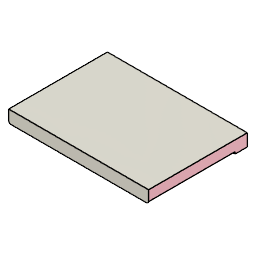
minecraft_pig (Autodesk Fusion 360 archive; units mm, degrees)
design "Bottom Face Plate"
part number: 2025-10-08-20-58-30-384
Autodesk Fusion 360 part; units mm, degrees
sketch "Bottom Face Plate" plane through (0, 0, 0) normal (0, 0, 1) x (1, 0, 0)
  line L0 (0, 0) -> (136, 0)
  line L1 (136, 0) -> (136, 96)
  line L2 (136, 96) -> (0, 96)
  line L3 (0, 96) -> (0, 0)
  dimension "d5" = 136
  dimension "d6" = 96
  constraint horizontal L0
  constraint vertical L1
  constraint horizontal L2
  constraint vertical L3
  constraint coincident L0.start L3.end
  measures "d5" distance of L0.start L0.end
  measures "d6" distance of L0.start L2.end
extrude "Extrude1" add sketch "Bottom Face Plate" along normal blind 12 makes body 1
ref_plane "WorkPlane1" through (68, 84, 6) normal (0, 1, 0) x (-1, 0, 0)
split "Split1" by plane through (68, 84, 6) normal (0, 1, 0) bodies 1 makes body 2 at (90.6667, 96, 8)
fillet "Fillet1" radius 2 2 edges at (136, 42, 0) (0, 42, 0) on bodies 1
combine "Combine2" operation add target body 1 tool bodies 2
equation "block_size = 16 mm" comment "The size of the blocks used for the dimensions of the Minecraft Pig."
equation "pine_thickness = 12 mm" comment "The thickness of the pine boards used for the Minecraft Pig's body."
equation "bottom_face_plate_length = 6 * block_size" comment "The length of the Bottom Face Plate that makes up the Minecraft Pig's face."
equation "bottom_face_plate_width = 10 * block_size - 2 * pine_thickness" comment "The width of the Bottom Face Plate that makes up the Minecraft Pig's face."
equation "d5 = bottom_face_plate_width"
equation "d6 = bottom_face_plate_length"
equation "d7 = pine_thickness"
equation "d9 = -pine_thickness"
equation "fillet_radius = 2 mm" comment "The radius of the fillets applied to the Bottom Face Plate."
equation "d12 = fillet_radius"
named bodies: "Bottom Face Plate", "Bottom Face Plate (1)"

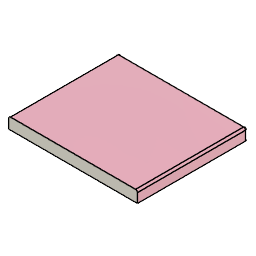
design "Top Face Plate"
part number: 2025-10-08-20-58-30-384
Autodesk Fusion 360 part; units mm, degrees
sketch "Top Face Plate" plane through (0, 0, 0) normal (0, 0, 1) x (1, 0, 0)
  line L0 (0, 0) -> (136, 0)
  line L1 (136, 0) -> (136, 116)
  line L2 (136, 116) -> (0, 116)
  line L3 (0, 116) -> (0, 0)
  dimension "d5" = 136
  dimension "d6" = 116
  constraint horizontal L0
  constraint vertical L1
  constraint horizontal L2
  constraint vertical L3
  constraint coincident L0.start L3.end
  measures "d5" distance of L0.start L0.end
  measures "d6" distance of L0.start L2.end
extrude "Extrude1" add sketch "Top Face Plate" along normal blind 12
fillet "Fillet1" radius 2 5 edges at (0, 58, 12) (136, 58, 12) (68, 116, 12) (136, 116, 6) (0, 116, 6)
equation "block_size = 16 mm" comment "The size of the blocks used for the dimensions of the Minecraft Pig."
equation "pine_thickness = 12 mm" comment "The thickness of the pine boards used for the Minecraft Pig's body."
equation "top_face_plate_length = 8 * block_size - pine_thickness" comment "The length of the Top Face Plate that makes up the Minecraft Pig's face."
equation "top_face_plate_width = 10 * block_size - 2 * pine_thickness" comment "The width of the Top Face Plate that makes up the Minecraft Pig's face."
equation "d5 = top_face_plate_width"
equation "d6 = top_face_plate_length"
equation "d7 = pine_thickness"
equation "fillet_radius = 2 mm" comment "The radius of the fillets applied to the Top Face Plate."
equation "d11 = fillet_radius"
named bodies: "Top Face Plate"

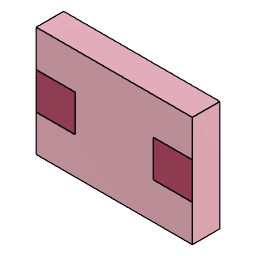
design "Nose Plate"
part number: 2025-10-11-08-44-41-819
Autodesk Fusion 360 part; units mm, degrees
sketch "Nose Plate" plane through (0, 0, 0) normal (0, 1, 0) x (1, 0, 0)
  line L0 (0, 0) -> (68, 0)
  line L1 (68, 0) -> (68, -48)
  line L2 (68, -48) -> (0, -48)
  line L3 (0, -48) -> (0, 0)
  dimension "d5" = 68
  dimension "d6" = 48
  constraint horizontal L0
  constraint vertical L1
  constraint horizontal L2
  constraint vertical L3
  constraint coincident L0.start L3.end
  measures "d5" distance of L0.start L0.end
  measures "d6" distance of L0.start L2.end
extrude "Extrude1" add sketch "Nose Plate" along normal blind 12 makes body 1
sketch "Nostrils" plane through (0, 0, 0) normal (0, -1, 0) x (1, 0, 0)
  line L0 (68, 48) -> (0, 48)
  line L1 (0, 48) -> (0, 0)
  line L2 (0, 0) -> (68, 0)
  line L3 (68, 0) -> (68, 48)
  line L4 (0, 32) -> (17, 32)
  line L5 (17, 32) -> (17, 16)
  line L6 (17, 16) -> (0, 16)
  line L7 (0, 16) -> (0, 32)
  line L8 (51, 32) -> (68, 32)
  line L9 (68, 32) -> (68, 16)
  line L10 (68, 16) -> (51, 16)
  line L11 (51, 16) -> (51, 32)
  dimension "d22" = 17
  dimension "d23" = 17
  dimension "d24" = 34
  dimension "d25" = 16
  dimension "d26" = 16
  dimension "d27" = 16
  dimension "d28" = 16
  constraint horizontal L4
  constraint vertical L5
  constraint horizontal L6
  constraint vertical L7
  constraint horizontal L8
  constraint vertical L9
  constraint horizontal L10
  constraint vertical L11
  constraint collinear L1 L7
  constraint collinear L3 L9
  measures "d22" distance of L4.start L4.end
  measures "d23" distance of L8.start L8.end
  measures "d24" distance of L5 L11
  measures "d25" distance of L4 L6
  measures "d26" distance of L8 L10
  measures "d27" distance of L0 L4
  measures "d28" distance of L0 L8
extrude "Extrude4" add sketch "Nostrils" along normal blind 0.01 separate body contours L3 L8 L9 L10 L11 | L1 L4 L5 L6 L7 makes body 2 at (5.6667, 0, 26.6667) makes body 3 at (56.6667, 0, 26.6667)
equation "block_size = 16 mm" comment "The size of the blocks used for the dimensions of the Minecraft Pig."
equation "pine_thickness = 12 mm" comment "The thickness of the pine boards used for the Minecraft Pig's body."
equation "nose_plate_height = 3 * block_size" comment "The height of the Nose Plate that makes up the Minecraft Pig's face."
equation "nose_plate_width = 4 * block_width" comment "The width of the Nose Plate that makes up the Minecraft Pig's face."
equation "d5 = nose_plate_width"
equation "d6 = nose_plate_height"
equation "d7 = pine_thickness"
equation "block_width = ( 10 * block_size - 2 * pine_thickness ) / 8" comment "The width of the blocks used for the nostrils of the Minecraft Pig."
equation "d22 = block_width"
equation "d23 = block_width"
equation "d25 = block_size"
equation "d26 = block_size"
equation "d27 = block_size"
equation "d28 = block_size"
named bodies: "Nose Plate", "Right Nostril", "Left Nostril"

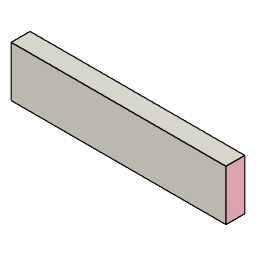
design "Back Face Plate"
part number: 2025-10-11-08-44-41-819
Autodesk Fusion 360 part; units mm, degrees
sketch "Back Face Plate" plane through (0, 0, 0) normal (0, 1, 0) x (1, 0, 0)
  line L0 (0, 0) -> (136, 0)
  line L1 (136, 0) -> (136, -32)
  line L2 (136, -32) -> (0, -32)
  line L3 (0, -32) -> (0, 0)
  dimension "d5" = 136
  dimension "d6" = 32
  constraint horizontal L0
  constraint vertical L1
  constraint horizontal L2
  constraint vertical L3
  constraint coincident L0.start L3.end
  measures "d5" distance of L0.start L0.end
  measures "d6" distance of L0.start L2.end
extrude "Extrude1" add sketch "Back Face Plate" along normal blind 12
equation "block_size = 16 mm" comment "The size of the blocks used for the dimensions of the Minecraft Pig."
equation "pine_thickness = 12 mm" comment "The thickness of the pine boards used for the Minecraft Pig's body."
equation "back_face_plate_height = 2 * block_size" comment "The height of the Back Face Plate that makes up the Minecraft Pig's face."
equation "back_face_plate_width = 10 * block_size - 2 * pine_thickness" comment "The width of the Back Face Plate that makes up the Minecraft Pig's face."
equation "d5 = back_face_plate_width"
equation "d6 = back_face_plate_height"
equation "d7 = pine_thickness"
equation "block_width = front_face_plate_width / 8" comment "The width of the blocks to use for the eyes of the Minecraft Pig."
equation "d10 = block_width"
equation "d11 = block_width"
equation "d12 = block_width"
equation "d13 = block_width"
equation "d14 = block_size"
equation "d15 = block_size"
equation "d16 = 3 * block_size"
equation "d17 = 3 * block_size"
named bodies: "Back Face Plate"

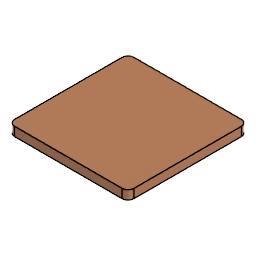
design "Felt Foot"
part number: 2025-10-02-09-28-42-821
Autodesk Fusion 360 part; units mm, degrees
sketch "Felt Foot" plane through (0, 0, 0) normal (0, 0, 1) x (1, 0, 0)
  line L0 (0, 0) -> (40, 0)
  line L1 (40, 0) -> (40, 40)
  line L2 (40, 40) -> (0, 40)
  line L3 (0, 40) -> (0, 0)
  dimension "d2" = 40
  dimension "d3" = 40
  constraint horizontal L0
  constraint vertical L1
  constraint horizontal L2
  constraint vertical L3
  constraint coincident L0.start L3.end
  measures "d2" distance of L0.start L2.end
  measures "d3" distance of L0.start L0.end
extrude "Extrude1" add sketch "Felt Foot" along normal blind 3
fillet "Fillet1" radius 2 4 edges at (0, 0, 1.5) (40, 0, 1.5) (40, 40, 1.5) (0, 40, 1.5)
equation "block_size = 16 mm" comment "The size of the blocks used for the dimensions of the Minecraft Pig."
equation "d2 = 2.5 * block_size"
equation "d3 = 2.5 * block_size"
equation "felt_thickness = 3 mm" comment "The thickness of the Felt Feet at the bottom of the Legs."
equation "d5 = felt_thickness"
equation "fillet_radius = 2 mm" comment "The radius of the fillets applied to the Felt Feet."
equation "d9 = fillet_radius"
named bodies: "Felt Foot"

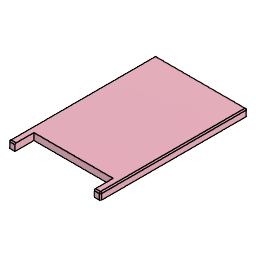
design "Top Plate"
part number: 2025-10-01-09-24-30-311
Autodesk Fusion 360 part; units mm, degrees
sketch "Top Plate" plane through (0, 0, 0) normal (0, 0, 1) x (1, 0, 0)
  line L0 (0, 0) -> (160, 0)
  line L1 (160, 0) -> (160, 256)
  line L2 (160, 256) -> (0, 256)
  line L3 (0, 256) -> (0, 0)
  line L4 (11, 0) -> (149, 0)
  line L5 (149, 0) -> (149, 33)
  line L6 (149, 33) -> (11, 33)
  line L7 (11, 33) -> (11, 0)
  dimension "d4" = 160
  dimension "d5" = 256
  dimension "d12" = 33
  dimension "d14" = 11
  dimension "d15" = 11
  constraint horizontal L0
  constraint vertical L1
  constraint horizontal L2
  constraint vertical L3
  constraint coincident L0.start L3.end
  constraint horizontal L4
  constraint vertical L5
  constraint horizontal L6
  constraint vertical L7
  constraint coincident L0 L4.start
  measures "d4" distance of L0.start L0.end
  measures "d5" distance of L0.end L1.end
  measures "d12" distance of L0 L6
  measures "d14" distance of L1 L5
  measures "d15" distance of L3 L7
extrude "Extrude1" add sketch "Top Plate" along normal blind 12 contours L0 L1 L2 L3 L5 L6 L7
fillet "Fillet2" radius 2 9 edges at (0, 0, 6) (160, 0, 6) (160, 256, 6) (0, 256, 6) (0, 128, 12) (80, 256, 12) (160, 128, 12) (5.5, 0, 12) (154.5, 0, 12)
equation "block_size = 16 mm" comment "The size of the blocks used for the dimensions of the Minecraft Pig."
equation "fillet_radius = 2 mm" comment "The radius of the fillets applied to the Top Plate."
equation "pine_thickness = 12 mm" comment "The thickness of the pine boards used for the Minecraft Pig's body."
equation "d4 = 10 * block_size"
equation "d5 = 16 * block_size"
equation "d6 = pine_thickness"
equation "tolerance = 1 mm" comment "The tolerance to add to the cutaway for the Minecraft Pig's face."
equation "cutaway_length = 2 * block_size + tolerance" comment "The length of the cutaway for the Minecraft Pig's face."
equation "d12 = cutaway_length"
equation "cutaway_side_width = pine_thickness - tolerance" comment "The width of the wood at the size of the cutaway for the Minecraft Pig's face."
equation "d14 = cutaway_side_width"
equation "d15 = cutaway_side_width"
equation "d17 = fillet_radius"
named bodies: "Top Plate"

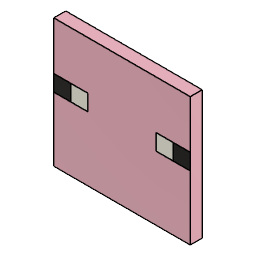
design "Front Face Plate"
part number: 2025-10-11-08-44-41-819
Autodesk Fusion 360 part; units mm, degrees
sketch "Front Face Plate" plane through (0, 0, 0) normal (0, 1, 0) x (1, 0, 0)
  line L0 (0, 0) -> (136, 0)
  line L1 (136, 0) -> (136, -128)
  line L2 (136, -128) -> (0, -128)
  line L3 (0, -128) -> (0, 0)
  dimension "d5" = 136
  dimension "d6" = 128
  constraint horizontal L0
  constraint vertical L1
  constraint horizontal L2
  constraint vertical L3
  constraint coincident L0.start L3.end
  measures "d5" distance of L0.start L0.end
  measures "d6" distance of L0.start L2.end
extrude "Extrude1" add sketch "Front Face Plate" along normal blind 12 makes body 1
sketch "Eyes" plane through (0, 0, 0) normal (0, -1, 0) x (1, 0, 0)
  line L0 (136, 128) -> (0, 128)
  line L1 (0, 128) -> (0, 0)
  line L2 (0, 0) -> (136, 0)
  line L3 (136, 0) -> (136, 128)
  line L4 (0, 80) -> (17, 80)
  line L5 (17, 80) -> (17, 64)
  line L6 (17, 64) -> (0, 64)
  line L7 (0, 64) -> (0, 80)
  line L8 (17, 80) -> (34, 80)
  line L9 (34, 80) -> (34, 64)
  line L10 (34, 64) -> (17, 64)
  line L11 (17, 64) -> (17, 80)
  line L12 (102, 80) -> (119, 80)
  line L13 (119, 80) -> (119, 64)
  line L14 (119, 64) -> (102, 64)
  line L15 (102, 64) -> (102, 80)
  line L16 (119, 80) -> (136, 80)
  line L17 (136, 80) -> (136, 64)
  line L18 (136, 64) -> (119, 64)
  line L19 (119, 64) -> (119, 80)
  dimension "d10" = 17
  dimension "d11" = 17
  dimension "d12" = 17
  dimension "d13" = 17
  dimension "d14" = 16
  dimension "d15" = 16
  dimension "d16" = 48
  dimension "d17" = 48
  constraint horizontal L4
  constraint vertical L5
  constraint horizontal L6
  constraint vertical L7
  constraint horizontal L8
  constraint vertical L9
  constraint horizontal L10
  constraint vertical L11
  constraint horizontal L12
  constraint vertical L13
  constraint horizontal L14
  constraint vertical L15
  constraint horizontal L16
  constraint vertical L17
  constraint horizontal L18
  constraint vertical L19
  constraint collinear L1 L7
  constraint collinear L3 L17
  constraint collinear L6 L10
  constraint collinear L14 L18
  measures "d10" distance of L4.start L4.end
  measures "d11" distance of L4.end L8.end
  measures "d12" distance of L12.start L12.end
  measures "d13" distance of L12.end L16.end
  measures "d14" distance of L8 L10
  measures "d15" distance of L12.start L14.end
  measures "d16" distance of L0 L4
  measures "d17" distance of L0 L16
extrude "Extrude2" add sketch "Eyes" along normal blind 0.01 separate body contours L3 L13 L16 L17 L18 L19 | L1 L4 L5 L6 L7 L11 makes body 2 at (5.6667, 0, 74.6667) makes body 3 at (124.6667, 0, 74.6667)
extrude "Extrude3" add sketch "Eyes" along normal blind 0.01 separate body contours L12 L13 L14 L15 L19 | L5 L8 L9 L10 L11 makes body 4 at (28.3333, 0, 69.3333) makes body 5 at (107.6667, 0, 69.3333)
equation "block_size = 16 mm" comment "The size of the blocks used for the dimensions of the Minecraft Pig."
equation "pine_thickness = 12 mm" comment "The thickness of the pine boards used for the Minecraft Pig's body."
equation "front_face_plate_height = 8 * block_size" comment "The height of the Front Face Plate that makes up the Minecraft Pig's face."
equation "front_face_plate_width = 10 * block_size - 2 * pine_thickness" comment "The width of the Front Face Plate that makes up the Minecraft Pig's face."
equation "d5 = front_face_plate_width"
equation "d6 = front_face_plate_height"
equation "d7 = pine_thickness"
equation "block_width = front_face_plate_width / 8" comment "The width of the blocks used for the eyes of the Minecraft Pig."
equation "d10 = block_width"
equation "d11 = block_width"
equation "d12 = block_width"
equation "d13 = block_width"
equation "d14 = block_size"
equation "d15 = block_size"
equation "d16 = 3 * block_size"
equation "d17 = 3 * block_size"
named bodies: "Front Face Plate", "Right Eye Pupil", "Left Eye Pupil", "Right Eye White", "Left Eye White"

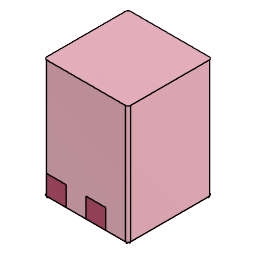
design "Front Leg"
part number: 2025-09-29-17-41-02-140
Autodesk Fusion 360 part; units mm, degrees
sketch "Leg" plane through (0, 0, 0) normal (0, 0, 1) x (1, 0, 0)
  line L0 (0, 0) -> (67, 0)
  line L1 (67, 0) -> (67, 67)
  line L2 (67, 67) -> (0, 67)
  line L3 (0, 67) -> (0, 0)
  dimension "d2" = 67
  dimension "d3" = 67
  constraint horizontal L0
  constraint vertical L1
  constraint horizontal L2
  constraint vertical L3
  constraint coincident L0.start L3.end
  measures "d2" distance of L0.start L0.end
  measures "d3" distance of L0.end L1.end
extrude "Extrude1" add sketch "Leg" along normal blind 96 makes body 1
sketch "Toes" plane through (0, 0, 0) normal (0, -1, 0) x (1, 0, 0)
  line L0 (0, 0) -> (67, 0)
  line L1 (67, 0) -> (67, 96)
  line L2 (67, 96) -> (0, 96)
  line L3 (0, 96) -> (0, 0)
  line L4 (2, 17.75) -> (17.75, 17.75)
  line L5 (17.75, 17.75) -> (17.75, 2)
  line L6 (17.75, 2) -> (2, 2)
  line L7 (2, 2) -> (2, 17.75)
  line L8 (33.5, 17.75) -> (49.25, 17.75)
  line L9 (49.25, 17.75) -> (49.25, 2)
  line L10 (49.25, 2) -> (33.5, 2)
  line L11 (33.5, 2) -> (33.5, 17.75)
  dimension "d16" = 15.75
  dimension "d17" = 15.75
  dimension "d18" = 15.75
  dimension "d19" = 2
  dimension "d20" = 2
  dimension "d21" = 15.75
  dimension "d22" = 17.75
  constraint horizontal L4
  constraint vertical L5
  constraint horizontal L6
  constraint vertical L7
  constraint horizontal L8
  constraint vertical L9
  constraint horizontal L10
  constraint vertical L11
  constraint collinear L6 L10
  constraint collinear L4 L8
  measures "d16" distance of L5.end L6.end
  measures "d17" distance of L9.end L10.end
  measures "d18" distance of L5 L11
  measures "d19" distance of L3 L7
  measures "d20" distance of L0 L6
  measures "d21" distance of L4.start L6.end
  measures "d22" distance of L1 L9
extrude "Extrude3" add sketch "Toes" along normal blind 0.01 separate body contours L4 L5 L6 L7 | L8 L9 L10 L11 makes body 2 at (7.25, 0, 7.25) makes body 3 at (38.75, 0, 7.25)
fillet "Fillet1" radius 2 8 edges at (0, 67, 48) (0, 33.5, 0) (0, 0, 48) (33.5, 0, 0) (67, 0, 48) (33.5, 67, 0) (67, 33.5, 0) (67, 67, 48) on bodies 1
equation "leg_width = 67 mm" comment "The dimensions of the 67 mm x 67 mm pine post used for the Legs."
equation "d2 = leg_width"
equation "d3 = leg_width"
equation "block_size = 16 mm" comment "The size of the blocks used for the dimensions of the Minecraft Pig."
equation "d5 = leg_height"
equation "fillet_radius = 2 mm" comment "The radius of the fillets applied to the Legs."
equation "d16 = toe_width"
equation "d17 = toe_width"
equation "d18 = toe_width"
equation "d19 = fillet_radius"
equation "d20 = fillet_radius"
equation "d21 = toe_width"
equation "d26 = fillet_radius"
equation "toe_width = ( leg_width - 2 * fillet_radius ) / 4" comment "The width and height of the two toes."
equation "leg_height = 6 * block_size" comment "The height of the Minecraft Pig's Legs."
named bodies: "Front Leg", "Right Toe", "Left Toe"

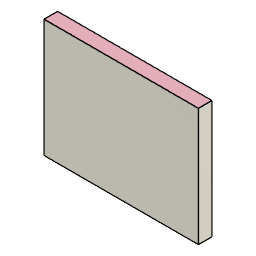
design "Back Plate"
part number: 2025-10-05-08-09-15-164
Autodesk Fusion 360 part; units mm, degrees
sketch "Back Plate" plane through (0, 0, 0) normal (0, 1, 0) x (1, 0, 0)
  line L0 (0, 0) -> (136, 0)
  line L1 (136, 0) -> (136, -104)
  line L2 (136, -104) -> (0, -104)
  line L3 (0, -104) -> (0, 0)
  dimension "d5" = 136
  dimension "d6" = 104
  constraint horizontal L0
  constraint vertical L1
  constraint horizontal L2
  constraint vertical L3
  constraint coincident L0.start L3.end
  measures "d5" distance of L0.start L0.end
  measures "d6" distance of L0.start L2.end
extrude "Extrude1" add sketch "Back Plate" along normal blind 12
equation "block_size = 16 mm" comment "The size of the blocks used for the dimensions of the Minecraft Pig."
equation "pine_thickness = 12 mm" comment "The thickness of the pine boards used for the Minecraft Pig's body."
equation "back_plate_height = 8 * block_size - 2 * pine_thickness" comment "The height of the Back Plate that makes up the Minecraft Pig's body."
equation "back_plate_width = 10 * block_size - 2 * pine_thickness" comment "The width of the Back Plate that makes up the Minecraft Pig's body."
equation "d5 = back_plate_width"
equation "d6 = back_plate_height"
equation "d7 = pine_thickness"
named bodies: "Back Plate"

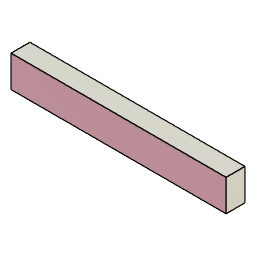
design "Front Plate"
part number: 2025-10-06-20-35-12-131
Autodesk Fusion 360 part; units mm, degrees
sketch "Front Plate" plane through (0, 0, 0) normal (0, 1, 0) x (1, 0, 0)
  line L0 (0, 0) -> (136, 0)
  line L1 (136, 0) -> (136, -20)
  line L2 (136, -20) -> (0, -20)
  line L3 (0, -20) -> (0, 0)
  dimension "d5" = 136
  dimension "d6" = 20
  constraint horizontal L0
  constraint vertical L1
  constraint horizontal L2
  constraint vertical L3
  constraint coincident L0.start L3.end
  measures "d5" distance of L0.start L0.end
  measures "d6" distance of L0.start L2.end
extrude "Extrude1" add sketch "Front Plate" along normal blind 12
equation "block_size = 16 mm" comment "The size of the blocks used for the dimensions of the Minecraft Pig."
equation "pine_thickness = 12 mm" comment "The thickness of the pine boards used for the Minecraft Pig's body."
equation "front_plate_height = 2 * block_size - 1 * pine_thickness" comment "The height of the Front Plate that makes up the Minecraft Pig's body."
equation "front_plate_width = 10 * block_size - 2 * pine_thickness" comment "The width of the Front Plate that makes up the Minecraft Pig's body."
equation "d5 = front_plate_width"
equation "d6 = front_plate_height"
equation "d7 = pine_thickness"
named bodies: "Front Plate"

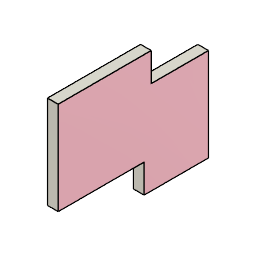
design "Left Side Face Plate"
part number: 2025-10-03-12-31-24-970
Autodesk Fusion 360 part; units mm, degrees
sketch "Side Face Plate" plane through (0, 0, 0) normal (1, 0, 0) x (0, 1, 0)
  line L0 (0, 0) -> (168, 0)
  line L1 (168, 0) -> (168, 136)
  line L2 (168, 136) -> (0, 136)
  line L3 (0, 136) -> (0, 0)
  line L4 (168, 136) -> (104, 136)
  line L5 (104, 136) -> (104, 104)
  line L6 (104, 104) -> (168, 104)
  line L7 (168, 104) -> (168, 136)
  line L8 (0, 0) -> (96, 0)
  line L9 (96, 0) -> (96, 32)
  line L10 (96, 32) -> (0, 32)
  line L11 (0, 32) -> (0, 0)
  dimension "d4" = 136
  dimension "d5" = 168
  dimension "d14" = 32
  dimension "d15" = 64
  dimension "d18" = 32
  dimension "d19" = 96
  constraint horizontal L0
  constraint vertical L1
  constraint horizontal L2
  constraint vertical L3
  constraint coincident L0.start L3.end
  constraint horizontal L4
  constraint vertical L5
  constraint horizontal L6
  constraint vertical L7
  constraint horizontal L8
  constraint vertical L9
  constraint horizontal L10
  constraint vertical L11
  measures "d4" distance of L0.start L2.end
  measures "d5" distance of L0.start L0.end
  measures "d14" distance of L4 L6
  measures "d15" distance of L5 L7
  measures "d18" distance of L8 L10
  measures "d19" distance of L9 L11
extrude "Extrude1" add sketch "Side Face Plate" along normal blind 12 contours L0 L1 L2 L3 L5 L6 L9 L10
equation "block_size = 16 mm" comment "The size of the blocks used for the dimensions of the Minecraft Pig."
equation "pine_thickness = 12 mm" comment "The thickness of the pine boards used for the Minecraft Pig's body."
equation "side_face_plate_height = 10 * block_size - 2 * pine_thickness" comment "The height of the Side Face Plates that make up the Minecraft Pig's face."
equation "d4 = side_face_plate_height"
equation "d5 = side_face_plate_length"
equation "d6 = pine_thickness"
equation "side_face_plate_length = ( 8 * block_size - 2 * pine_thickness ) + 4 * block_size" comment "The length of the Side Face Plates that make up the Minecraft Pig's face."
equation "top_cutaway_height = 2 * block_size" comment "The height of the top cutaway in the Side Face Plates."
equation "top_cutaway_length = 4 * block_size" comment "The length of the top cutaway in the Side Face Plates."
equation "d14 = top_cutaway_height"
equation "d15 = top_cutaway_length"
equation "bottom_cutaway_height = 2 * block_size" comment "The height of the bottom cutaway in the Side Face Plates."
equation "bottom_cutaway_length = 6 * block_size" comment "The length of the bottom cutaway in the Side Face Plates."
equation "d18 = bottom_cutaway_height"
equation "d19 = bottom_cutaway_length"
named bodies: "Left Side Face Plate"

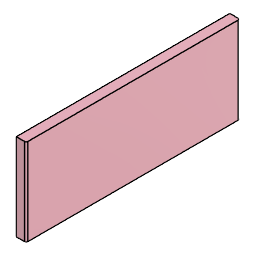
design "Side Plate"
part number: 2025-10-03-12-31-24-970
Autodesk Fusion 360 part; units mm, degrees
sketch "Side Plate" plane through (0, 0, 0) normal (1, 0, 0) x (0, 1, 0)
  line L0 (0, 0) -> (256, 0)
  line L1 (256, 0) -> (256, 104)
  line L2 (256, 104) -> (0, 104)
  line L3 (0, 104) -> (0, 0)
  dimension "d4" = 104
  dimension "d5" = 256
  constraint horizontal L0
  constraint vertical L1
  constraint horizontal L2
  constraint vertical L3
  constraint coincident L0.start L3.end
  measures "d4" distance of L0.start L2.end
  measures "d5" distance of L0.start L0.end
extrude "Extrude1" add sketch "Side Plate" along normal blind 12
fillet "Fillet1" radius 2 2 edges at (12, 0, 52) (12, 256, 52)
equation "block_size = 16 mm" comment "The size of the blocks used for the dimensions of the Minecraft Pig."
equation "pine_thickness = 12 mm" comment "The thickness of the pine boards used for the Minecraft Pig's body."
equation "side_plate_height = 8 * block_size - 2 * pine_thickness" comment "The height of the Side Plates that make up the Minecraft Pig's body."
equation "d4 = side_plate_height"
equation "d5 = 16 * block_size"
equation "d6 = pine_thickness"
equation "fillet_radius = 2 mm" comment "The radius of the fillets applied to the Side Plates."
equation "d10 = fillet_radius"
named bodies: "Side Plate"

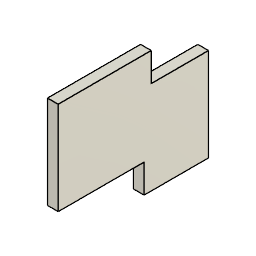
design "Right Side Face Plate"
part number: 2025-10-03-12-31-24-970
Autodesk Fusion 360 part; units mm, degrees
sketch "Side Face Plate" plane through (0, 0, 0) normal (1, 0, 0) x (0, 1, 0)
  line L0 (0, 0) -> (168, 0)
  line L1 (168, 0) -> (168, 136)
  line L2 (168, 136) -> (0, 136)
  line L3 (0, 136) -> (0, 0)
  line L4 (168, 136) -> (104, 136)
  line L5 (104, 136) -> (104, 104)
  line L6 (104, 104) -> (168, 104)
  line L7 (168, 104) -> (168, 136)
  line L8 (0, 0) -> (96, 0)
  line L9 (96, 0) -> (96, 32)
  line L10 (96, 32) -> (0, 32)
  line L11 (0, 32) -> (0, 0)
  dimension "d4" = 136
  dimension "d5" = 168
  dimension "d14" = 32
  dimension "d15" = 64
  dimension "d18" = 32
  dimension "d19" = 96
  constraint horizontal L0
  constraint vertical L1
  constraint horizontal L2
  constraint vertical L3
  constraint coincident L0.start L3.end
  constraint horizontal L4
  constraint vertical L5
  constraint horizontal L6
  constraint vertical L7
  constraint horizontal L8
  constraint vertical L9
  constraint horizontal L10
  constraint vertical L11
  measures "d4" distance of L0.start L2.end
  measures "d5" distance of L0.start L0.end
  measures "d14" distance of L4 L6
  measures "d15" distance of L5 L7
  measures "d18" distance of L8 L10
  measures "d19" distance of L9 L11
extrude "Extrude1" add sketch "Side Face Plate" along normal blind 12 contours L0 L1 L2 L3 L5 L6 L9 L10
equation "block_size = 16 mm" comment "The size of the blocks used for the dimensions of the Minecraft Pig."
equation "pine_thickness = 12 mm" comment "The thickness of the pine boards used for the Minecraft Pig's body."
equation "side_face_plate_height = 10 * block_size - 2 * pine_thickness" comment "The height of the Side Face Plates that make up the Minecraft Pig's face."
equation "d4 = side_face_plate_height"
equation "d5 = side_face_plate_length"
equation "d6 = pine_thickness"
equation "side_face_plate_length = ( 8 * block_size - 2 * pine_thickness ) + 4 * block_size" comment "The length of the Side Face Plates that make up the Minecraft Pig's face."
equation "top_cutaway_height = 2 * block_size" comment "The height of the top cutaway in the Side Face Plates."
equation "top_cutaway_length = 4 * block_size" comment "The length of the top cutaway in the Side Face Plates."
equation "d14 = top_cutaway_height"
equation "d15 = top_cutaway_length"
equation "bottom_cutaway_height = 2 * block_size" comment "The height of the bottom cutaway in the Side Face Plates."
equation "bottom_cutaway_length = 6 * block_size" comment "The length of the bottom cutaway in the Side Face Plates."
equation "d18 = bottom_cutaway_height"
equation "d19 = bottom_cutaway_length"
named bodies: "Right Side Face Plate"
